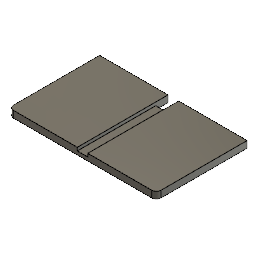
verstärkung (Autodesk Fusion 360 design; units mm, degrees)
Autodesk Fusion 360 part; units mm, degrees
sketch "Skizze1" plane through (0, 0, 0) normal (0, 1, 0) x (1, 0, 0)
  line L0 (32.5, 20) -> (-32.5, 20)
  line L1 (-32.5, 20) -> (-32.5, -20)
  line L2 (-32.5, -20) -> (32.5, -20)
  line L3 (32.5, -20) -> (32.5, 20)
  line L4 (32.5, 20) -> (-32.5, -20) construction
  line L5 (-32.5, 20) -> (32.5, -20) construction
  dimension "d1" = 40
  dimension "d2" = 65
  constraint horizontal L0
  constraint perpendicular L0 L1
  constraint parallel L0 L2
  constraint parallel L1 L3
  constraint coincident L4 origin
  constraint coincident L5 origin
  measures "d1" distance of L0.end L1.end
  measures "d2" distance of L1.end L2.end
extrude "Extrusion1" add sketch "Skizze1" along normal blind 3
sketch "Skizze2" plane through (0, 3, 0) normal (0, 1, 0) x (-1, 0, 0)
  line L0 (-32.5, 20) -> (-32.5, -20)
  line L1 (-32.5, -20) -> (32.5, -20)
  line L2 (32.5, -20) -> (32.5, 20)
  line L3 (32.5, 20) -> (-32.5, 20)
  line L4 (2.3, -20) -> (-2.3, -20)
  line L5 (-2.3, -20) -> (-2.3, -14.5)
  line L6 (-2.3, -14.5) -> (2.3, -14.5)
  line L7 (2.3, -14.5) -> (2.3, -20)
  line L8 (2.3, -20) -> (-2.3, -14.5) construction
  line L9 (-2.3, -20) -> (2.3, -14.5) construction
  point P0 (0, -17.25)
  dimension "d5" = 4.6
  dimension "d6" = 5.5
  constraint horizontal L4
  constraint perpendicular L4 L5
  constraint parallel L4 L6
  constraint parallel L5 L7
  constraint coincident L1 L4.start
  constraint coincident L8 P0
  constraint coincident L9 P0
  constraint vertical origin P0
  measures "d5" distance of L5.end L6.end
  measures "d6" distance of L4.end L5.end
extrude "Extrusion2" cut sketch "Skizze2" against normal blind 3 contours L1 L4 L5 L6 L7
sketch "Skizze3" plane through (0, 3, 0) normal (0, 1, 0) x (-1, 0, 0)
  line L0 (2.3, -14.5) -> (2.3, -20)
  line L1 (2.3, -20) -> (32.5, -20)
  line L2 (32.5, -20) -> (32.5, 20)
  line L3 (32.5, 20) -> (-32.5, 20)
  line L4 (-32.5, 20) -> (-32.5, -20)
  line L5 (-32.5, -20) -> (-2.3, -20)
  line L6 (-2.3, -20) -> (-2.3, -14.5)
  line L7 (-2.3, -14.5) -> (2.3, -14.5)
  line L8 (2.3, -14.5) -> (-2.3, -14.5)
  line L9 (-2.3, -14.5) -> (-2.3, 20)
  line L10 (-2.3, 20) -> (2.3, 20)
  line L11 (2.3, 20) -> (2.3, -14.5)
  constraint horizontal L8
  constraint vertical L9
  constraint horizontal L10
  constraint vertical L11
  constraint coincident L3 L9.end
  constraint coincident L0.start L7.end
  constraint collinear L6 L9
extrude "Extrusion3" cut sketch "Skizze3" against normal blind 1.4 contours L3 L7 L8 L9 L10 L11
fillet "Abrundung1" radius 2 2 edges at (-32.5, 1.5, 20) (32.5, 1.5, 20)
